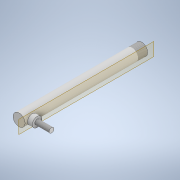
# Autodesk Inventor part: stav
Saved by Autodesk Inventor 2021 (Build 250183000, 183)
## iProperties
Created: 2021-02-09
Part Number: stav
Material: Generic
Document SubType Name: Modeling
Designer: marcu
Density: 1 g/cm^3
Appearance: Default
Author: marcu
Autodesk Inventor part; units mm, degrees
ref_plane "XZ Plane" through (0, 0, 0) normal (0, 1, 0) x (-1, 0, 0)
ref_plane "XY Plane" through (0, 0, 0) normal (0, 0, 1) x (1, 0, 0)
sketch "Sketch1" plane through (0, 0, 0) normal (0, 0, 1) x (1, 0, 0)
  circle A0 centre (0, 0) radius 12.5
  dimension "d0" = 25
  constraints: 1 centre point, 1 coincident
  measures "d0" diameter of A0
extrude "Extrusion1" add sketch "Sketch1" along normal blind 255
thread "Thread1" size "M25x2" class "6g" standard "ISO Metric profile" length 20
ref_plane "Work Plane1" through (12.5, 0, 0) normal (1, 0, 0) x (0, 1, 0)
sketch "Sketch2" plane through (12.5, 0, 0) normal (1, 0, 0) x (0, 1, 0)
  circle A0 centre (0, 240) radius 10
  line L0 (12.5, 255) -> (-12.5, 255) projected
  point P0 (0, 0)
  dimension "d5" = 20
  dimension "d6" = 15
  dimension "d16" = 12.5
  constraints: 1 centre point
  measures "d5" diameter of A0
  measures "d6" distance from line of L0 A0.centre
  measures "d16" horizontal distance of L0.start A0.centre
extrude "Extrusion2" add sketch "Sketch2" along normal blind 10
sketch "Sketch3" plane through (22.5, 0, 240) normal (1, 0, 0) x (0, 0, -1)
  arc A0 (10, 0) -> (-10, 0) centre (0, 0) ccw projected
  circle A1 centre (0, 0) radius 5
  point P0 (240, 0)
  dimension "d11" = 10
  constraints: 1 centre point, 1 coincident
  measures "d11" diameter of A1
extrude "Extrusion3" add sketch "Sketch3" along normal blind 30
thread "Thread3" size "M10x1.5" class "6g" standard "ANSI Metric M Profile" full length
body "Solid1"
